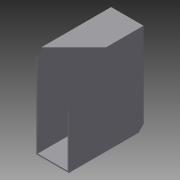
# Autodesk Inventor part: Case
Saved by Autodesk Inventor 2014 (Build 180170000, 170)
## iProperties
Created: 2014-08-29
Part Number: Case
Material: Generic
Document SubType Name: Modeling
Designer: sam
Density: 1 g/cm^3
Appearance: Default
Author: sam
Autodesk Inventor part; units mm, degrees
ref_plane "YZ Plane" through (0, 0, 0) normal (1, 0, 0) x (0, 1, 0)
ref_plane "XZ Plane" through (0, 0, 0) normal (0, 1, 0) x (-1, 0, 0)
ref_plane "Work Plane1" through (5, 0, 0) normal (1, 0, 0) x (0, 1, 0)
sketch "Sketch1" plane through (5, 0, 0) normal (1, 0, 0) x (0, 1, 0)
  line L0 (-72.5, 60) -> (72.5, 60)
  line L1 (72.5, 60) -> (72.5, -60)
  line L2 (72.5, -60) -> (-72.5, -60)
  line L3 (-72.5, -60) -> (-72.5, 60)
  line L4 (-72.5, 60) -> (72.5, -60) construction
  line L5 (72.5, 60) -> (-72.5, -60) construction
  point P0 (0, 0)
  dimension "d0" = 145
  dimension "d1" = 120
  constraints: 12 end point, 2 midpoint, 2 parallel, 1 horizontal, 1 perpendicular
  measures "d0" distance of L1.end L2.end
  measures "d1" distance of L0.end L1.end
extrude "Extrusion1" add sketch "Sketch1" along normal blind 49
shell "Shell2" thickness 2 removed faces 1 at (21.3333, -24.1667, 60)
body "Solid1"
